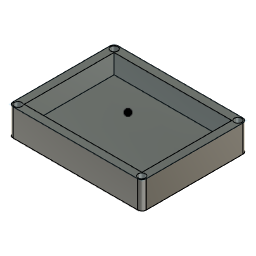
_part_1.318b750a-d903-4d5c-bca3-ea630c4a2858 (Autodesk Fusion 360 design; units mm, degrees)
Autodesk Fusion 360 part; units mm, degrees
sketch "Sketch1" plane through (0, 0, 0) normal (0, 0, 1) x (1, 0, 0) in component "part 1"
  line L0 (-15.5, 12.25) -> (15.5, 12.25)
  line L1 (15.5, 12.25) -> (15.5, -12.25)
  line L2 (15.5, -12.25) -> (-15.5, -12.25)
  line L3 (-15.5, -12.25) -> (-15.5, 12.25)
  line L4 (-15.5, 12.25) -> (15.5, -12.25) construction
  line L5 (15.5, 12.25) -> (-15.5, -12.25) construction
  dimension "d1" = 31
  dimension "d2" = 24.5
  constraint horizontal L0
  constraint perpendicular L0 L1
  constraint parallel L0 L2
  constraint parallel L1 L3
  constraint coincident L4 origin
  constraint coincident L5 origin
  measures "d1" distance of L0.start L0.end
  measures "d2" distance of L0.start L2.end
extrude "Extrude1" add sketch "Sketch1" along normal blind 6.3 in component "part 1"
sketch "Sketch2" plane through (0, 0, 6.3) normal (0, 0, 1) x (-1, 0, 0) in component "part 1"
  line L0 (15.5, 12.25) -> (-15.5, 12.25)
  line L1 (-15.5, 12.25) -> (-15.5, -12.25)
  line L2 (-15.5, -12.25) -> (15.5, -12.25)
  line L3 (15.5, -12.25) -> (15.5, 12.25)
shell "Shell1" thickness 1.8 removed faces 1 at (-5.1667, 4.0833, 6.3) in component "part 1"
sketch "Sketch3" plane through (0, 0, 6.3) normal (0, 0, 1) x (-1, 0, 0) in component "part 1"
  circle A0 centre (14.4, -11.2) radius 0.85
  line L0 (0, 0) -> (0, -3.5)
  line L1 (0, 0) -> (3.5, 0)
  circle A1 centre (-14.4, -11.2) radius 0.85
  circle A2 centre (-14.4, 11.2) radius 0.85
  circle A3 centre (14.4, 11.2) radius 0.85
  dimension "d8" = 1.7
  dimension "d9" = 11.2
  dimension "d10" = 14.4
  constraint coincident L0.start L1.start
  constraint vertical L0
  constraint perpendicular L0 L1
  constraint symmetric A0 L0 A1
  constraint symmetric A0 L1 A3
  constraint symmetric L1 A1 A2
  measures "d8" diameter of A0
  measures "d9" vertical distance of L0.start A0.centre
  measures "d10" horizontal distance of L0.start A0.centre
extrude "Extrude2" cut sketch "Sketch3" against normal blind 4 in component "part 1"
fillet "Fillet1" radius 1 1 edges at (15.5, -12.25, 3.15) in component "part 1"
fillet "Fillet1" radius 1 1 edges at (15.5, 12.25, 3.15) in component "part 1"
fillet "Fillet1" radius 1 1 edges at (-15.5, 12.25, 3.15) in component "part 1"
fillet "Fillet1" radius 1 1 edges at (-15.5, -12.25, 3.15) in component "part 1"
component "part 1" placed x (1, 0, 0) y (0, 1, 0) z (0, 0, 1) at (0, 0, 0)
